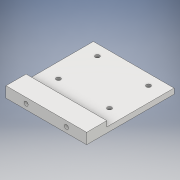
# Autodesk Inventor part: 앞뒷면PSD받침대
Saved by Autodesk Inventor 2017 (Build 210142000, 142)
## iProperties
Part Number: 앞뒷면PSD받침대
Material: ABS 플라스틱
Document SubType Name: Modeling
Designer: minom
Mass: 20.2156 g
Surface Area: 94.9651 cm^2
Volume: 19.0713 cm^3
Density: 1.06 g/cm^3
Appearance: 매끄러움 - 흰색
Author: minom
Autodesk Inventor part; units mm, degrees
ref_plane "YZ Plane" through (0, 0, 0) normal (1, 0, 0) x (0, 1, 0)
ref_plane "XZ Plane" through (0, 0, 0) normal (0, 1, 0) x (-1, 0, 0)
ref_plane "XY Plane" through (0, 0, 0) normal (0, 0, 1) x (1, 0, 0)
sketch "스케치1" plane through (0, 0, 0) normal (0, 0, 1) x (1, 0, 0)
  line L0 (0, 0) -> (60, 0)
  line L1 (60, 0) -> (60, 70)
  line L2 (60, 70) -> (0, 70)
  line L3 (0, 70) -> (0, 0)
  dimension "d0" = 60
  dimension "d1" = 70
  constraints: 8 end point, 2 parallel, 1 horizontal, 1 perpendicular
  measures "d0" distance of L2.end L1.end
  measures "d1" distance of L1.end L0.end
extrude "돌출1" add sketch "스케치1" along normal blind 8
sketch "스케치2" plane through (0, 0, 8) normal (0, 0, 1) x (1, 0, 0)
  line L0 (0, 0) -> (60, 0) projected
  line L1 (60, 0) -> (60, 70) projected
  line L2 (60, 70) -> (0, 70) projected
  line L3 (0, 70) -> (0, 0) projected
  line L4 (60, 0) -> (60, 70) projected
  line L5 (0, 70) -> (60, 70)
  line L6 (60, 70) -> (60, 20)
  line L7 (60, 20) -> (0, 20)
  line L8 (0, 20) -> (0, 70)
  constraints: 8 end point, 2 parallel, 1 horizontal, 1 perpendicular, 1 point on line
extrude "돌출2" cut sketch "스케치2" against normal blind 4 contours L3 L2 L1 L7
sketch "스케치3" plane through (0, 0, 4) normal (0, 0, 1) x (1, 0, 0)
  line L0 (60, 70) -> (60, 20) projected
  line L1 (0, 70) -> (60, 70) projected
  line L2 (0, 20) -> (0, 70) projected
  line L3 (60, 20) -> (0, 20) projected
  line L4 (60, 70) -> (0, 70) projected
  circle A0 centre (11, 62) radius 1.6
  circle A1 centre (49, 62) radius 1.6
  circle A2 centre (11, 33) radius 1.6
  circle A3 centre (49, 33) radius 1.6
  point P0 (0, 0)
  dimension "d8" = 3.2
  dimension "d9" = 3.2
  dimension "d14" = 3.2
  dimension "d15" = 3.2
  dimension "d16" = 11
  dimension "d17" = 8
  dimension "d18" = 8
  dimension "d19" = 11
  dimension "d20" = 29
  dimension "d21" = 11
  dimension "d22" = 11
  dimension "d23" = 29
  constraints: 4 centre point
  measures "d8" diameter of A0
  measures "d9" diameter of A1
  measures "d14" diameter of A2
  measures "d15" diameter of A3
  measures "d16" distance from line of L2 A0.centre
  measures "d17" distance from line of L1 A0.centre
  measures "d18" distance from line of L1 A1.centre
  measures "d19" distance from line of L0 A1.centre
  measures "d20" distance of A1.centre A3.centre
  measures "d21" distance from line of L0 A3.centre
  measures "d22" distance from line of L2 A2.centre
  measures "d23" distance of A0.centre A2.centre
extrude "돌출3" cut sketch "스케치3" against normal blind 4 contours A0 | A1 | A2 | A3
sketch "스케치4" plane through (0, 0, 0) normal (0, -1, 0) x (1, 0, 0)
  line L0 (0, 0) -> (60, 0) projected
  line L1 (60, 0) -> (60, 8) projected
  line L2 (0, 8) -> (60, 8) projected
  line L3 (0, 0) -> (0, 8) projected
extrude "돌출4" cut sketch "스케치4" against normal blind 5
sketch "스케치5" plane through (0, 5, 0) normal (0, -1, 0) x (1, 0, 0)
  circle A0 centre (15, 4) radius 1.5
  circle A1 centre (45, 4) radius 1.5
  line L0 (60, 0) -> (0, 0) projected
  line L1 (0, 8) -> (60, 8) projected
  line L2 (0, 0) -> (0, 8) projected
  line L3 (60, 8) -> (60, 0) projected
  dimension "d24" = 3
  dimension "d25" = 3
  dimension "d26" = 4
  dimension "d27" = 4
  dimension "d28" = 15
  dimension "d29" = 15
  constraints: 2 centre point
  measures "d24" diameter of A0
  measures "d25" diameter of A1
  measures "d26" distance from line of L0 A0.centre
  measures "d27" distance from line of L1 A1.centre
  measures "d28" distance from line of L2 A0.centre
  measures "d29" distance from line of L3 A1.centre
extrude "돌출5" cut sketch "스케치5" against normal blind 8 contours A0 | A1
